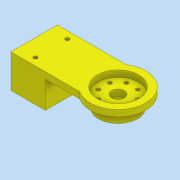
# Autodesk Inventor part: motor_6809_ab
Saved by Autodesk Inventor 2020.2 (Build 242310000, 310)
## iProperties
Created: 2016-12-03
Part Number: motor_6809_ab
Material: Allgemein
Document SubType Name: Modeling
Designer: paulg
Density: 1 g/cm^3
Appearance: Vorgabe
Author: paulg
Autodesk Inventor part; units mm, degrees
ref_plane "YZ Plane" through (0, 0, 0) normal (1, 0, 0) x (0, 1, 0)
ref_plane "XZ Plane" through (0, 0, 0) normal (0, 1, 0) x (-1, 0, 0)
ref_plane "XY Plane" through (0, 0, 0) normal (0, 0, 1) x (1, 0, 0)
sketch "Sketch1" plane through (0, 0, 0) normal (0, 0, 1) x (1, 0, 0)
  circle A0 centre (0, 0) radius 15.1
  circle A1 centre (0, 0) radius 5
  dimension "d0" = 30.2
  dimension "d1" = 10
  constraints: 2 centre point, 2 coincident
  measures "d0" diameter of A0
  measures "d1" diameter of A1
extrude "Extrusion1" add sketch "Sketch1" along normal blind 8
sketch "Sketch3" plane through (0, 0, 8) normal (0, 0, 1) x (1, 0, 0)
  circle A0 centre (0, 0) radius 5 projected
  circle A1 centre (0, 0) radius 15.1 projected
  circle A2 centre (0, 0) radius 16.1
  dimension "d21" = 1
  constraints: 1 centre point, 1 coincident
  measures "d21" radial gap between concentric circles of A1 A2
extrude "Extrusion3" add sketch "Sketch3" along normal blind 1 contours A1 | A2
sketch "Sketch4" plane through (0, 0, 9) normal (0, 0, 1) x (1, 0, 0)
  circle A0 centre (0, 0) radius 5 projected
  circle A1 centre (0, 0) radius 16.1 projected
  line L0 (0, 0) -> (-41.1674, 0) construction
  line L1 (-65, -18) -> (-11.758, -18)
  line L2 (-11.758, 18) -> (-65, 18)
  line L3 (-65, 18) -> (-65, -18)
  line L4 (-11.758, 18) -> (-11.758, -18) construction
  line L5 (0, 0) -> (-51.0801, 0) construction
  line L6 (-38.379, 18) -> (-38.379, -18)
  circle A2 centre (-51.6895, 12.375) radius 1.5
  circle A3 centre (-51.6895, -12.375) radius 1.5
  circle A4 centre (0, 0) radius 6
  circle A5 centre (0, 0) radius 9
  line L7 (-51.6895, 12.375) -> (-51.6895, -12.375) construction
  arc A6 (-11.7222, 18.0234) -> (-11.758, 18) centre (0, 0) ccw
  arc A7 (-11.758, -18) -> (-11.758, 18) centre (0, 0) ccw
  point P0 (-38.379, 0.051)
  point P1 (-51.6895, 0)
  point P2 (-11.758, -18)
  point P3 (-11.7222, 18.0234)
  dimension "d29" = 0
  dimension "d30" = 36
  dimension "d31" = 65
  dimension "d494" = 0
  dimension "d629" = 3
  dimension "d630" = 24.75
  dimension "d633" = 12
  dimension "d634" = 3
  dimension "d646" = 21.5
  constraints: 16 end point, 6 centre point, 6 point on line, 5 coincident, 4 perpendicular, 4 point on circle, 3 horizontal, 3 midpoint, 2 vertical, 1 equal radius, 1 parallel, 9 other
  measures "d30" distance between parallel lines of L1 L2
  measures "d31" distance from line of A0.centre L3
  measures "d494" distance between parallel lines of L0 L5
  measures "d629" diameter of A2
  measures "d630" distance of A3.centre A2.centre
  measures "d633" diameter of A4
  measures "d634" radial gap between concentric circles of A5 A4
  measures "d646" radius of A7
extrude "Extrusion5" add sketch "Sketch4" along normal blind 5 contours L3 L2 L6 L1 | L6 L2 A6 A7 L1
extrude "Extrusion86" add sketch "Sketch4" against normal blind 21 contours L3 L2 L6 L1
extrude "Extrusion87" cut sketch "Sketch4" along normal blind 4 from surface at -9 contours A0 | A4
sketch "Skizze97" plane through (0, 0, 0) normal (0, 0, 1) x (1, 0, 0)
  circle A0 centre (0, 0) radius 5
  circle A1 centre (0, 0) radius 22.6
  line L0 (0, 0) -> (0, -22.6) construction
  circle A2 centre (0, 0) radius 22.6
  line L1 (0, 0) -> (-8.6486, -20.8797) construction
  circle A3 centre (-4.4965, -10.8556) radius 1.5
  dimension "d637" = 22.5
  dimension "d638" = 3
  dimension "d639" = 11.75
  constraints: 4 centre point, 4 end point, 4 point on circle, 1 coincident, 1 point on line, 1 vertical
  measures "d637" angle of L1 L0
  measures "d638" diameter of A3
  measures "d639" distance of A0.centre A3.centre
extrude "Extrusion88" cut sketch "Skizze97" along normal through all contours A3
pattern_circular "Runde Anordnung5" count 8 over 360 about axis through (0, 0, -10) along (0, 0, 1) of "Extrusion88"
equation "\"E_\" = 1"
equation "\"Rr_\" = 2"
equation "\"R_\" = 19"
equation "\"Ri\" = 11.75"
equation "\"Ra\" = 21.5"
equation "\"Rl\" = 17.5"
equation "\"Rla\" = 18.5"
equation "\"Rli\" = 15"
equation "\"Rsi\" = 5"
equation "\"Rsa\" = 7.5"
equation "\"Rca\" = 7"
equation "\"Ras\" = 1"
equation "\"Rci\" = 5"
equation "\"Rea\" = 3.5"
equation "\"Rei\" = 2"
body "Solid1"
